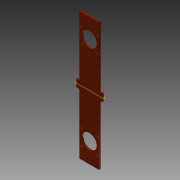
# Autodesk Inventor part: Panel4_FanCutout
Saved by Autodesk Inventor 2015 (Build 190159000, 159)
## iProperties
Created: 2014-08-06
Part Number: Panel4_FanCutout
Material: Wood (Oak)
Document SubType Name: Modeling
Designer: Patrick Camilleri
Density: 0.76 g/cm^3
Appearance: White Oak - Natural Medium Gloss
Author: Patrick Camilleri
Autodesk Inventor part; units mm, degrees
ref_plane "YZ Plane" through (0, 0, 0) normal (1, 0, 0) x (0, 1, 0)
ref_plane "XZ Plane" through (0, 0, 0) normal (0, 1, 0) x (-1, 0, 0)
sketch "Sketch1" plane through (0, 0, 0) normal (0, 1, 0) x (-1, 0, 0)
  line L0 (20, 129.3) -> (-20, 129.3)
  line L1 (-20, 129.3) -> (-20, -129.3)
  line L2 (-20, -129.3) -> (20, -129.3)
  line L3 (20, -129.3) -> (20, 129.3)
  line L4 (20, 129.3) -> (-20, -129.3) construction
  line L5 (-20, 129.3) -> (20, -129.3) construction
  line L6 (23, 132.3) -> (-23, 132.3) construction
  line L7 (-23, 132.3) -> (-23, -132.3) construction
  line L8 (-23, -132.3) -> (23, -132.3) construction
  line L9 (23, -132.3) -> (23, 132.3) construction
  line L10 (26, 7.5) -> (20, 7.5)
  line L11 (20, 7.5) -> (20, -7.5)
  line L12 (20, -7.5) -> (26, -7.5)
  line L13 (26, -7.5) -> (26, 7.5)
  line L14 (26, 7.5) -> (20, -7.5) construction
  line L15 (20, 7.5) -> (26, -7.5) construction
  line L16 (-20, 7.5) -> (-26, 7.5)
  line L17 (-26, 7.5) -> (-26, -7.5)
  line L18 (-26, -7.5) -> (-20, -7.5)
  line L19 (-20, -7.5) -> (-20, 7.5)
  line L20 (-20, 7.5) -> (-26, -7.5) construction
  line L21 (-26, 7.5) -> (-20, -7.5) construction
  point P0 (0, 0)
  point P1 (23, 0)
  point P2 (-23, 0)
  point P3 (0, 0)
  dimension "d0" = 40
  dimension "d1" = 258.6
  dimension "d2" = 3
  dimension "d3" = 15
  dimension "d18" = 6
  dimension "d19" = 15
  constraints: 44 end point, 9 midpoint, 8 parallel, 4 perpendicular, 3 horizontal, 1 point on line, 3 other
  measures "d0" distance of L2.end L1.end
  measures "d1" distance of L1.end L0.end
  measures "d2" distance between parallel lines of L3 L9
  measures "d3" distance of L11.end L10.end
  measures "d18" distance of L18.end L17.end
  measures "d19" distance of L17.end L16.end
extrude "Extrusion1" add sketch "Sketch1" along normal blind 3
sketch "Sketch3" plane through (0, 0, 0) normal (0, -1, 0) x (1, 0, 0)
  line L0 (-20, 129.3) -> (20, 129.3) projected
  line L1 (-16, 105.3) -> (16, 105.3) construction
  line L2 (16, 105.3) -> (16, 73.3) construction
  line L3 (16, 73.3) -> (-16, 73.3) construction
  line L4 (-16, 73.3) -> (-16, 105.3) construction
  line L5 (-16, 105.3) -> (16, 73.3) construction
  line L6 (16, 105.3) -> (-16, 73.3) construction
  point P0 (0, 0)
  point P1 (0, 89.3)
  dimension "d69" = 32
  dimension "d70" = 32
  dimension "d71" = 40
  constraints: 12 end point, 2 midpoint, 2 parallel, 1 coincident, 1 horizontal, 1 perpendicular
  measures "d69" distance of L2.end L3.end
  measures "d70" distance of L1.end L2.end
  measures "d71" distance from line of point (0, 89.3) L0
hole "Hole2" at (16, 0, 105.3) direction (0, 1, 0) diameter 5 end through all
pattern_linear "Rectangular Pattern1" count 2 spacing 32 along (-1, 0, 0) count 2 spacing 32 along (0, 0, -1) of "Hole2"
sketch "Sketch5" plane through (0, 0, 0) normal (0, -1, 0) x (1, 0, 0)
  circle A0 centre (16, 73.3) radius 2.5 projected
  circle A1 centre (-16, 105.3) radius 2.5 projected
  line L0 (-16, 105.3) -> (16, 73.3) construction
  circle A2 centre (0, 89.3) radius 15
  point P0 (0, 0)
  dimension "d86" = 30
  constraints: 2 end point, 1 centre point, 1 midpoint
  measures "d86" diameter of A2
extrude "Extrusion4" cut sketch "Sketch5" against normal through all contours A2
mirror "Mirror2" about plane through (0, 0, 0) normal (0, 0, 1) of "Extrusion4", "Hole2", "Rectangular Pattern1"
body "Solid1"
